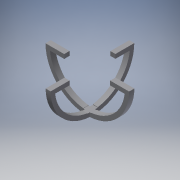
# Autodesk Inventor part: SentiBot botton
Saved by Autodesk Inventor 2016 (Build 200138000, 138)
## iProperties
Created: 2015-07-02
Part Number: SentiBot botton
Material: Generic
Document SubType Name: Modeling
Designer: Sudhar
Density: 1 g/cm^3
Appearance: Default
Author: Sudhar
Autodesk Inventor part; units mm, degrees
ref_plane "YZ Plane" through (0, 0, 0) normal (1, 0, 0) x (0, 1, 0)
ref_plane "XZ Plane" through (0, 0, 0) normal (0, 1, 0) x (-1, 0, 0)
ref_plane "XY Plane" through (0, 0, 0) normal (0, 0, 1) x (1, 0, 0)
sketch "Sketch1" plane through (0, 0, 0) normal (0, 0, 1) x (1, 0, 0)
  arc A0 (-2.9756, -24.1911) -> (22.4244, 1.2089) centre (-2.9756, 1.2089) ccw
  line L0 (-2.9756, 1.2089) -> (-2.9756, -24.1911)
  line L1 (-2.9756, 1.2089) -> (22.4244, 1.2089)
  dimension "d0" = 50.8
  constraints: 4 end point, 2 point on circle, 1 centre point, 1 perpendicular, 1 vertical
  measures "d0" diameter of A0
revolve "Revolution1" add sketch "Sketch1" angle 360 about axis through (-2.9756, 1.2089, 0) along (0, -1, 0)
sketch "Sketch3" plane through (0, 0, 0) normal (0, 0, 1) x (1, 0, 0)
  line L0 (-2.7068, 20.711) -> (-2.7068, -36.5415)
  constraints: 2 end point, 1 vertical
shell "Shell1" thickness 2.54 removed faces 0
sketch "Sketch6" plane through (-2.9756, 1.2089, 0) normal (0, 1, 0) x (1, 0, 0)
  line L0 (-38.7778, 26.1829) -> (-1.5476, 26.1829)
  line L1 (-1.5476, 26.1829) -> (-1.5476, 1.5658)
  line L2 (-1.5476, 1.5658) -> (-38.7778, 1.5658)
  line L3 (-38.7778, 1.5658) -> (-38.7778, 26.1829)
  line L4 (-38.7778, -1.6527) -> (-1.5476, -1.6527)
  line L5 (-1.5476, -1.6527) -> (-1.5476, -31.924)
  line L6 (-1.5476, -31.924) -> (-38.7778, -31.924)
  line L7 (-38.7778, -31.924) -> (-38.7778, -1.6527)
  line L8 (1.4969, 26.1829) -> (35.2476, 26.1829)
  line L9 (35.2476, 26.1829) -> (35.2476, 1.5658)
  line L10 (35.2476, 1.5658) -> (1.4969, 1.5658)
  line L11 (1.4969, 1.5658) -> (1.4969, 26.1829)
  line L12 (35.2476, -1.6527) -> (1.4969, -1.6527)
  line L13 (1.4969, -1.6527) -> (1.4969, -32.6199)
  line L14 (1.4969, -32.6199) -> (35.2476, -32.6199)
  line L15 (35.2476, -32.6199) -> (35.2476, -1.6527)
  point P0 (2.9756, 0)
  constraints: 32 end point, 8 parallel, 7 point on line, 4 horizontal, 4 perpendicular
extrude "Extrusion4" cut sketch "Sketch6" against normal blind 25.4
sketch "Sketch7" plane through (-1.4788, -1.3311, -1.5658) normal (0, -1, 0) x (1, 0, 0)
  line L0 (21.1614, 3.2185) -> (0, 3.2185) projected
  line L1 (0, 3.2185) -> (-3.0445, 3.2185)
  line L2 (-3.0445, 3.2185) -> (-3.0445, 0)
  line L3 (-3.0445, 0) -> (0, 0)
  line L4 (0, 0) -> (0, 3.2185)
  point P0 (1.4788, 1.5658)
  constraints: 8 end point, 2 parallel, 1 horizontal, 1 perpendicular
extrude "Extrusion5" add sketch "Sketch7" along normal blind 22.86
sketch "Sketch8" plane through (-1.4788, 1.2089, -1.5658) normal (0, 1, 0) x (1, 0, 0)
  circle A0 centre (-1.5514, -1.5658) radius 13.97
  point P0 (1.4788, -1.5658)
  dimension "d38" = 27.94
  constraints: 1 centre point
  measures "d38" diameter of A0
extrude "Extrusion6" cut sketch "Sketch8" against normal blind 10.16
sketch "Sketch9" plane through (-1.4788, -8.9511, -1.5658) normal (0, 1, 0) x (1, 0, 0)
  line L0 (-3.9499, 1.7048) -> (0.9942, 1.7048)
  line L1 (0.9942, 1.7048) -> (0.9942, -4.633)
  line L2 (0.9942, -4.633) -> (-3.9499, -4.633)
  line L3 (-3.9499, -4.633) -> (-3.9499, 1.7048)
  point P0 (1.4788, -1.5658)
  constraints: 8 end point, 2 parallel, 1 horizontal, 1 perpendicular
extrude "Extrusion7" cut sketch "Sketch9" against normal blind 12.7
body "Solid1"
